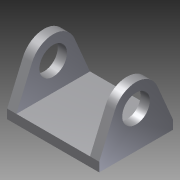
# Autodesk Inventor part: manipulator pnumaitic pivot
Saved by Autodesk Inventor 2012 (Build 160160000, 160)
## iProperties
Created: 2013-09-04
Part Number: manipulator pnumaitic pivot
Material: Default
Document SubType Name: Modeling
Designer: Bryce
Density: 1 g/cm^3
Author: Bryce
Autodesk Inventor part; units mm, degrees
ref_plane "YZ Plane" through (0, 0, 0) normal (1, 0, 0) x (0, 1, 0)
ref_plane "XZ Plane" through (0, 0, 0) normal (0, 1, 0) x (-1, 0, 0)
ref_plane "XY Plane" through (0, 0, 0) normal (0, 0, 1) x (1, 0, 0)
sketch "Sketch1" plane through (0, 0, 0) normal (0, 0, 1) x (1, 0, 0)
  line L0 (0, 0) -> (31.75, 0)
  line L1 (31.75, 0) -> (31.75, 25.4)
  line L2 (0, 25.4) -> (0, 0)
  line L3 (28.575, 25.4) -> (28.575, 3.175)
  line L4 (28.575, 3.175) -> (3.175, 3.175)
  line L5 (3.175, 3.175) -> (3.175, 25.4)
  line L6 (31.75, 25.4) -> (28.575, 25.4)
  line L7 (3.175, 25.4) -> (0, 25.4)
  dimension "d0" = 25.4
  dimension "d1" = 31.75
  dimension "d2" = 3.175
  dimension "d3" = 3.175
  dimension "d4" = 3.175
  constraints: 16 end point, 4 parallel, 1 collinear, 1 horizontal, 1 perpendicular
  measures "d0" distance of L2.start L0.start
  measures "d1" distance of L0.start L0.end
  measures "d2" distance between parallel lines of L2 L5
  measures "d3" distance between parallel lines of L4 L0
  measures "d4" distance between parallel lines of L1 L3
extrude "Extrusion1" add sketch "Sketch1" along normal blind 25.4
sketch "Sketch2" plane through (31.75, 0, 0) normal (1, 0, 0) x (0, 0, -1)
  line L0 (-25.4, 25.4) -> (-25.4, 0) projected
  line L1 (0, 0) -> (-25.4, 0) projected
  line L2 (0, 0) -> (0, 25.4) projected
  line L3 (0, 25.4) -> (-25.4, 25.4) projected
  circle A0 centre (-12.7, 12.7) radius 4.7625
  arc A1 (-5.4006, 15.818) -> (-19.9994, 15.818) centre (-12.7, 12.7) ccw
  line L4 (-19.9994, 15.818) -> (-25.4, 3.175)
  line L5 (-5.4006, 15.818) -> (0, 3.175)
  point P0 (0, 12.7)
  dimension "d9" = 9.525
  dimension "d13" = 3.175
  dimension "d14" = 12.7
  dimension "d15" = 7.9375
  dimension "d16" = 12.7
  constraints: 4 end point, 2 centre point, 2 point on circle, 2 point on line, 2 tangent, 1 concentric, 1 horizontal alignment, 1 midpoint
  measures "d9" diameter of A0
  measures "d13" distance from line of L1 L4.end
  measures "d14" distance from line of L1 A0.centre
  measures "d15" radius of A1
  measures "d16" distance from line of L0 A0.centre
extrude "Extrusion2" cut sketch "Sketch2" against normal through all contours L3 L2 L5 A1 L4 L0 | A0
equation "\"d3\" = d2"
equation "\"d4\" = d3"
body "Solid1"
